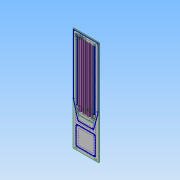
# Autodesk Inventor part: Ply back
Saved by Autodesk Inventor 2013 (Build 170138000, 138)
## iProperties
Created: 2018-07-07
Part Number: Ply back
Material: Generic
Document SubType Name: Modeling
Designer: Jeff Vyduna
Density: 1 g/cm^3
Author: Jeff Vyduna
Autodesk Inventor part; units mm, degrees
ref_plane "YZ Plane" through (0, 0, 0) normal (1, 0, 0) x (0, 1, 0)
ref_plane "XZ Plane" through (0, 0, 0) normal (0, 1, 0) x (-1, 0, 0)
ref_plane "XY Plane" through (0, 0, 0) normal (0, 0, 1) x (1, 0, 0)
sketch "TwoLineColumn" plane through (0, 0, 0) normal (0, 0, 1) x (1, 0, 0)
  line L0 (50.8, -550.7609) -> (50.8, 922.4391) construction
  line L1 (101.6, -550.7609) -> (101.6, 922.4391) construction
  arc A0 (101.6, 922.4391) -> (50.8, 922.4391) centre (76.2, 922.4391) ccw construction
  arc A1 (101.6, -550.7609) -> (152.4, -550.7609) centre (127, -550.7609) ccw construction
  line L2 (56.896, -550.7609) -> (56.896, 922.4391)
  arc A2 (95.504, 922.4391) -> (56.896, 922.4391) centre (76.2, 922.4391) ccw
  line L3 (95.504, 922.4391) -> (95.504, -550.7609)
  arc A3 (95.504, -550.7609) -> (158.496, -550.7609) centre (127, -550.7609) ccw
  line L4 (44.704, -550.7609) -> (44.704, 922.4391)
  arc A4 (107.696, 922.4391) -> (44.704, 922.4391) centre (76.2, 922.4391) ccw
  line L5 (107.696, 922.4391) -> (107.696, -550.7609)
  arc A5 (107.696, -550.7609) -> (146.304, -550.7609) centre (127, -550.7609) ccw
  line L6 (50.8, -550.7609) -> (152.4, -550.7609) construction
  dimension "d4" = 1473.2
  dimension "lineSpacing" = 50.8
  dimension "d6" = 25.4
  dimension "d9" = 6.096
  dimension "d10" = 6.096
  measures "d4" distance of L0.start L0.end
  measures "lineSpacing" distance between parallel lines of L1 L0
  measures "d6" radius of A1
  measures "d9" distance between parallel lines of L1 L3
  measures "d10" distance between parallel lines of L5 L1
sketch "TwoLineColumnEnd" plane through (0, 0, 0) normal (0, 0, 1) x (1, 0, 0)
  line L0 (103.0524, -741.9843) -> (103.0524, 731.2157)
  arc A0 (166.0444, 731.2157) -> (103.0524, 731.2157) centre (134.5484, 731.2157) ccw
  line L1 (166.0444, 731.2157) -> (166.0444, -741.9843)
  line L2 (109.1484, -741.9843) -> (109.1484, 731.2157) construction
  line L3 (159.9484, -741.9843) -> (159.9484, 731.2157) construction
  arc A1 (159.9484, 731.2157) -> (109.1484, 731.2157) centre (134.5484, 731.2157) ccw construction
  line L4 (115.2444, -741.9843) -> (115.2444, 731.2157)
  arc A2 (153.8524, 731.2157) -> (115.2444, 731.2157) centre (134.5484, 731.2157) ccw
  line L5 (153.8524, 731.2157) -> (153.8524, -741.9843)
  line L6 (109.1484, -741.9843) -> (159.9484, -741.9843) construction
  dimension "d22" = 1473.2
  dimension "d23" = 50.8
  dimension "d25" = 6.096
  dimension "d26" = 6.096
  dimension "d29" = 50.8
  measures "d22" distance of L2.start L2.end
  measures "d23" distance between parallel lines of L3 L2
  measures "d25" distance between parallel lines of L3 L5
  measures "d26" distance between parallel lines of L1 L3
  measures "d29" distance of L2.start L6.end
sketch "15mm Neon profile" plane through (0, 0, 0) normal (0, 0, 1) x (1, 0, 0)
  circle A0 centre (522.6685, 24.7098) radius 6.985 construction
  line L0 (516.6995, 21.082) -> (528.6375, 21.082) construction
  line L1 (528.6375, 21.082) -> (528.6375, 6.35) construction
  line L2 (528.6375, 6.35) -> (516.6995, 6.35) construction
  line L3 (516.6995, 6.35) -> (516.6995, 21.082) construction
  point P0 (522.6685, 16.011)
  dimension "d73" = 13.97
  dimension "d74" = 11.938
  dimension "d76" = 14.732
  measures "d73" diameter of A0
  measures "d74" distance of L0.start L0.end
  measures "d76" distance of L0.end L1.end
sketch "U Bolt hole and bore" plane through (0, 0, 0) normal (0, 0, 1) x (1, 0, 0)
  circle A0 centre (40.0435, 30.4025) radius 9.525
  circle A1 centre (74.9685, 30.4025) radius 9.525
  circle A2 centre (40.0435, 30.4025) radius 3.9688
  circle A3 centre (74.9685, 30.4025) radius 3.9688
  point P0 (68.2625, 33.02)
  dimension "d100" = 19.05
  dimension "d102" = 34.925
  dimension "d105" = 7.9375
  measures "d100" diameter of A0
  measures "d102" distance of A1.centre A0.centre
  measures "d105" diameter of A2
sketch "Stock" plane through (0, 0, 0) normal (0, 0, 1) x (1, 0, 0)
  line L0 (0, 0) -> (604.8375, 0)
  line L1 (604.8375, 0) -> (604.8375, 2438.4)
  line L2 (604.8375, 2438.4) -> (0, 2438.4)
  line L3 (0, 2438.4) -> (0, 0)
  dimension "d1" = 604.8375
  dimension "d2" = 2438.4
  constraints: 8 end point, 2 parallel, 1 coincident, 1 horizontal, 1 perpendicular
  measures "d1" distance of L2.end L1.end
  measures "d2" distance of L1.end L0.end
extrude "Stock Extrusion" add sketch "Stock" along normal blind 19.05
sketch "LEDPocket" plane through (0, 0, 19.05) normal (0, 0, 1) x (1, 0, 0)
  line L0 (0, 0) -> (604.8375, 0) projected
  line L1 (604.8375, 0) -> (604.8375, 2438.4) projected
  line L2 (63.5, 120.65) -> (63.5, 0) construction
  line L3 (541.3375, 2438.4) -> (541.3375, 0) construction
  line L4 (68.5882, 922.2642) -> (113.2243, 755.68)
  line L5 (137.7589, 736.854) -> (467.0786, 736.854)
  line L6 (491.6132, 755.68) -> (536.2493, 922.2642)
  line L7 (80.7802, 923.8693) -> (108.8317, 819.18)
  line L8 (133.3662, 800.354) -> (471.4713, 800.354)
  line L9 (496.0058, 819.18) -> (524.0573, 923.8693)
  line L10 (474.1227, 844.55) -> (474.1227, 2317.75)
  arc A0 (537.1147, 2317.75) -> (474.1227, 2317.75) centre (505.6187, 2317.75) ccw
  line L11 (537.1147, 2317.75) -> (537.1147, 928.8382)
  line L12 (480.2187, 844.55) -> (480.2187, 2317.75) construction
  line L13 (531.0187, 844.55) -> (531.0187, 2317.75) construction
  arc A1 (531.0187, 2317.75) -> (480.2187, 2317.75) centre (505.6187, 2317.75) ccw construction
  line L14 (486.3147, 844.55) -> (486.3147, 2317.75)
  arc A2 (524.9227, 2317.75) -> (486.3147, 2317.75) centre (505.6187, 2317.75) ccw
  line L15 (524.9227, 2317.75) -> (524.9227, 930.4433)
  line L16 (480.2187, 844.55) -> (531.0187, 844.55) construction
  line L17 (67.7227, 928.8382) -> (67.7228, 2317.75)
  arc A3 (130.7148, 2317.75) -> (67.7228, 2317.75) centre (99.2188, 2317.75) ccw
  line L18 (130.7148, 2317.75) -> (130.7147, 844.55)
  arc A4 (130.7147, 844.55) -> (169.3227, 844.55) centre (150.0187, 844.55) ccw
  line L19 (73.8187, 844.55) -> (73.8188, 2317.75) construction
  line L20 (124.6187, 844.55) -> (124.6188, 2317.75) construction
  arc A5 (124.6188, 2317.75) -> (73.8188, 2317.75) centre (99.2188, 2317.75) ccw construction
  arc A6 (124.6187, 844.55) -> (175.4187, 844.55) centre (150.0187, 844.55) ccw construction
  line L21 (79.9147, 930.4433) -> (79.9147, 2317.75)
  arc A7 (118.5228, 2317.75) -> (79.9147, 2317.75) centre (99.2188, 2317.75) ccw
  line L22 (118.5228, 2317.75) -> (118.5227, 844.55)
  arc A8 (118.5227, 844.55) -> (181.5147, 844.55) centre (150.0187, 844.55) ccw
  line L23 (73.8187, 844.55) -> (175.4187, 844.55) construction
  line L24 (169.3227, 844.55) -> (169.3228, 2317.75)
  arc A9 (232.3148, 2317.75) -> (169.3228, 2317.75) centre (200.8188, 2317.75) ccw
  line L25 (232.3148, 2317.75) -> (232.3147, 844.55)
  arc A10 (232.3147, 844.55) -> (270.9227, 844.55) centre (251.6187, 844.55) ccw
  line L26 (175.4187, 844.55) -> (175.4188, 2317.75) construction
  line L27 (226.2187, 844.55) -> (226.2188, 2317.75) construction
  arc A11 (226.2188, 2317.75) -> (175.4188, 2317.75) centre (200.8188, 2317.75) ccw construction
  arc A12 (226.2187, 844.55) -> (277.0187, 844.55) centre (251.6187, 844.55) ccw construction
  line L28 (181.5147, 844.55) -> (181.5148, 2317.75)
  arc A13 (220.1227, 2317.75) -> (181.5148, 2317.75) centre (200.8188, 2317.75) ccw
  line L29 (220.1227, 2317.75) -> (220.1227, 844.55)
  arc A14 (220.1227, 844.55) -> (283.1147, 844.55) centre (251.6187, 844.55) ccw
  line L30 (270.9227, 844.55) -> (270.9228, 2317.75)
  arc A15 (333.9148, 2317.75) -> (270.9228, 2317.75) centre (302.4187, 2317.75) ccw
  line L31 (333.9148, 2317.75) -> (333.9147, 844.55)
  arc A16 (333.9147, 844.55) -> (372.5227, 844.55) centre (353.2187, 844.55) ccw
  line L32 (277.0187, 844.55) -> (277.0188, 2317.75) construction
  line L33 (327.8187, 844.55) -> (327.8188, 2317.75) construction
  arc A17 (327.8188, 2317.75) -> (277.0188, 2317.75) centre (302.4187, 2317.75) ccw construction
  arc A18 (327.8187, 844.55) -> (378.6187, 844.55) centre (353.2187, 844.55) ccw construction
  line L34 (283.1147, 844.55) -> (283.1148, 2317.75)
  arc A19 (321.7228, 2317.75) -> (283.1148, 2317.75) centre (302.4187, 2317.75) ccw
  line L35 (321.7228, 2317.75) -> (321.7227, 844.55)
  arc A20 (321.7227, 844.55) -> (384.7148, 844.55) centre (353.2187, 844.55) ccw
  line L36 (372.5227, 844.55) -> (372.5228, 2317.75)
  arc A21 (435.5147, 2317.75) -> (372.5228, 2317.75) centre (404.0188, 2317.75) ccw
  line L37 (435.5147, 2317.75) -> (435.5147, 844.55)
  arc A22 (435.5147, 844.55) -> (474.1227, 844.55) centre (454.8187, 844.55) ccw
  line L38 (378.6187, 844.55) -> (378.6188, 2317.75) construction
  line L39 (429.4187, 844.55) -> (429.4187, 2317.75) construction
  arc A23 (429.4187, 2317.75) -> (378.6188, 2317.75) centre (404.0188, 2317.75) ccw construction
  arc A24 (429.4187, 844.55) -> (480.2187, 844.55) centre (454.8187, 844.55) ccw construction
  line L40 (384.7148, 844.55) -> (384.7148, 2317.75)
  arc A25 (423.3227, 2317.75) -> (384.7148, 2317.75) centre (404.0188, 2317.75) ccw
  line L41 (423.3227, 2317.75) -> (423.3228, 844.55)
  arc A26 (423.3228, 844.55) -> (486.3147, 844.55) centre (454.8187, 844.55) ccw
  arc A27 (67.7227, 928.8382) -> (68.5882, 922.2642) centre (93.1227, 928.8382) ccw
  arc A28 (79.9147, 930.4433) -> (80.7802, 923.8693) centre (105.3147, 930.4433) ccw
  arc A29 (108.8317, 819.18) -> (133.3662, 800.354) centre (133.3662, 825.754) ccw
  arc A30 (471.4713, 800.354) -> (496.0058, 819.18) centre (471.4713, 825.754) ccw
  arc A31 (524.0573, 923.8693) -> (524.9227, 930.4433) centre (499.5227, 930.4433) ccw
  arc A32 (536.2493, 922.2642) -> (537.1147, 928.8382) centre (511.7147, 928.8382) ccw
  arc A33 (467.0786, 736.854) -> (491.6132, 755.68) centre (467.0786, 762.254) ccw
  arc A34 (113.2243, 755.68) -> (137.7589, 736.854) centre (137.7589, 762.254) ccw
  point P0 (0, 2438.4)
  point P1 (67.7227, 925.4942)
  point P2 (537.1147, 925.4942)
  point P3 (79.9147, 927.0993)
  point P4 (524.9227, 927.0993)
  point P5 (113.8761, 800.354)
  point P6 (490.9614, 800.354)
  point P7 (118.2687, 736.854)
  point P8 (486.5687, 736.854)
  point P9 (302.4187, 736.854)
  point P10 (302.4187, 800.354)
  dimension "d7" = 73.8187
  dimension "d18" = 63.5
  dimension "d19" = 120.65
  dimension "d20" = 2438.4
  dimension "d21" = 541.3375
  dimension "d32" = 63.5
  dimension "d33" = 44.196
  dimension "d38" = 844.55
  dimension "d41" = 1473.2
  dimension "d42" = 50.8
  dimension "d43" = 6.096
  dimension "d44" = 6.096
  dimension "d45" = 50.8
  dimension "d49" = 1473.2
  dimension "d50" = 50.8
  dimension "d51" = 25.4
  dimension "d52" = 6.096
  dimension "d53" = 6.096
  dimension "d89" = 120.65
  dimension "d166" = 368.3
  dimension "d167" = 12.192
  dimension "d168" = 25.4
  dimension "d171" = 12.192
  dimension "d172" = 165
  constraints: 80 end point, 70 point on circle, 40 tangent, 35 centre point, 24 vertical, 21 parallel, 16 point on line, 13 equal radius, 12 horizontal alignment, 2 midpoint, 2 perpendicular, 2 vertical alignment, 1 coincident, 1 horizontal, 9 other
  measures "d7" distance from line of L19 point (0, 0)
  measures "d18" distance from line of point (0, 0) L2
  measures "d19" distance of L2.start L2.end
  measures "d20" distance of L3.start L3.end
  measures "d21" distance from line of L0.start L3
  measures "d32" distance between parallel lines of L5 L8
  measures "d33" distance from line of L19.start L8
  measures "d38" distance from line of L19.start L0
  measures "d41" distance of L12.start L12.end
  measures "d42" distance between parallel lines of L13 L12
  measures "d43" distance between parallel lines of L13 L15
  measures "d44" distance between parallel lines of L11 L13
  measures "d45" distance of L12.start L16.end
  measures "d49" distance of L19.start L19.end
  measures "d50" distance between parallel lines of L20 L19
  measures "d51" radius of A6
  measures "d52" distance between parallel lines of L20 L22
  measures "d53" distance between parallel lines of L18 L20
  measures "d89" vertical distance of A3.centre point (0, 2438.4)
  measures "d166" distance of point (118.269, 736.854) point (486.569, 736.854)
  measures "d167" distance between parallel lines of L4 L7
  measures "d168" radius of A27
  measures "d171" distance between parallel lines of L6 L9
  measures "d172" angle of L7 L21
extrude "Main rope pocket" cut sketch "LEDPocket" against normal blind 12.7
sketch "Side profile reference" plane through (0, 0, 0) normal (0, -1, 0) x (1, 0, 0)
  line L0 (0, 0) -> (604.8375, 0) projected
  line L1 (604.8375, 0) -> (604.8375, 19.05) projected
  line L2 (0, 19.05) -> (604.8375, 19.05) projected
  line L3 (0, 0) -> (0, 19.05) projected
  line L4 (598.4875, 38.1) -> (586.2955, 38.1) construction
  line L5 (586.2955, 38.1) -> (586.2955, 25.4) construction
  line L6 (586.2955, 25.4) -> (598.4875, 25.4) construction
  line L7 (598.4875, 25.4) -> (598.4875, 38.1) construction
  line L8 (604.8375, 19.05) -> (541.3375, 19.05) construction
  line L9 (541.3375, 19.05) -> (541.3375, 38.1) construction
  line L10 (541.3375, 38.1) -> (604.8375, 38.1) construction
  line L11 (604.8375, 38.1) -> (604.8375, 19.05) construction
  line L12 (547.6875, 38.1) -> (573.0875, 38.1) construction
  line L13 (573.0875, 38.1) -> (573.0875, 40.64) construction
  line L14 (573.0875, 40.64) -> (547.6875, 40.64) construction
  line L15 (547.6875, 40.64) -> (547.6875, 38.1) construction
  line L16 (579.4375, 40.64) -> (516.6995, 40.64) construction
  line L17 (516.6995, 40.64) -> (516.6995, 45.847) construction
  line L18 (516.6995, 45.847) -> (579.4375, 45.847) construction
  line L19 (579.4375, 45.847) -> (579.4375, 40.64) construction
  circle A0 centre (522.6685, 24.7098) radius 6.985 construction
  line L20 (516.6995, 21.082) -> (528.6375, 21.082) construction
  line L21 (528.6375, 21.082) -> (528.6375, 6.35) construction
  line L22 (528.6375, 6.35) -> (516.6995, 6.35) construction
  line L23 (516.6995, 6.35) -> (516.6995, 21.082) construction
  circle A1 centre (592.3915, 43.7598) radius 6.985 construction
  line L24 (586.4225, 40.132) -> (598.3605, 40.132) construction
  line L25 (598.3605, 40.132) -> (598.3605, 25.4) construction
  line L26 (598.3605, 25.4) -> (586.4225, 25.4) construction
  line L27 (586.4225, 25.4) -> (586.4225, 40.132) construction
  point P0 (566.7375, 19.05)
  point P1 (592.3915, 25.4)
  point P2 (592.3915, 25.4)
  dimension "d75" = 12.7
  dimension "d80" = 12.192
  dimension "d88" = 6.35
  dimension "d90" = 63.5
  dimension "d91" = 19.05
  dimension "d92" = 25.4
  dimension "d93" = 2.54
  dimension "d94" = 6.35
  dimension "d95" = 12.7
  dimension "d96" = 6.35
  dimension "d97" = 5.207
  dimension "d98" = 0
  dimension "d99" = 12.7
  constraints: 32 end point, 8 parallel, 5 horizontal, 4 perpendicular, 1 coincident, 1 collinear, 1 midpoint, 1 point on line, 1 other
  measures "d80" distance of L6.end L5.end
  measures "d88" horizontal distance of L1.end L6.end
  measures "d90" distance of L9.end L10.end
  measures "d91" distance of L8.end L9.end
  measures "d92" distance of L14.end L13.end
  measures "d93" distance of L13.end L12.end
  measures "d94" distance of L9.end L12.start
  measures "d96" horizontal distance of L16.start L12.end
  measures "d97" distance of L16.end L17.end
  measures "d99" vertical distance of L10.end L6.end
sketch "U-Bolt holes" plane through (0, 0, 19.05) normal (0, 0, 1) x (1, 0, 0)
  line L0 (0, 0) -> (604.8375, 0) projected
  line L1 (604.8375, 0) -> (604.8375, 2438.4) projected
  line L2 (0, 2438.4) -> (0, 0) projected
  line L3 (604.8375, 2438.4) -> (0, 2438.4) projected
  point P0 (53.975, 33.02)
  point P1 (88.9, 33.02)
  point P2 (515.9375, 33.02)
  point P3 (550.8625, 33.02)
  point P4 (531.8125, 2365.375)
  point P5 (496.8875, 2365.375)
  point P6 (73.025, 2365.375)
  point P7 (107.95, 2365.375)
  dimension "d109" = 33.02
  dimension "d110" = 34.925
  dimension "d111" = 34.925
  dimension "d112" = 19.05
  dimension "d113" = 53.975
  dimension "d114" = 53.975
  dimension "d115" = 34.925
  dimension "d116" = 34.925
  dimension "d117" = 19.05
  dimension "d126" = 73.025
  constraints: 6 horizontal alignment
  measures "d109" distance from line of L0 point (53.975, 33.02)
  measures "d110" distance of point (88.9, 33.02) point (53.975, 33.02)
  measures "d111" distance of point (550.862, 33.02) point (515.937, 33.02)
  measures "d112" horizontal distance of point (53.975, 33.02) point (73.025, 2365.375)
  measures "d113" distance from line of L1 point (550.862, 33.02)
  measures "d114" distance from line of L2 point (53.975, 33.02)
  measures "d115" distance of point (73.025, 2365.375) point (107.95, 2365.375)
  measures "d116" distance of point (531.812, 2365.375) point (496.887, 2365.375)
  measures "d117" horizontal distance of point (531.812, 2365.375) point (550.862, 33.02)
  measures "d126" distance from line of L3 point (73.025, 2365.375)
hole "Hole1" at (73.025, 2365.375, 19.05) at (107.95, 2365.375, 19.05) at (496.8875, 2365.375, 19.05) at (531.8125, 2365.375, 19.05) at (550.8625, 33.02, 19.05) at (515.9375, 33.02, 19.05) at (88.9, 33.02, 19.05) at (53.975, 33.02, 19.05) direction (0, 0, -1) diameter 7.9375 end through all counterbore diameter 19.05 counterbore depth 6.35
ref_plane "Work Plane1" through (0, 0, 6.35) normal (0, 0, 1) x (1, 0, 0)
sketch "WeatherProof panel" plane through (0, 0, 6.35) normal (0, 0, 1) x (1, 0, 0)
  line L0 (524.9228, 801.1635) -> (524.9227, 2317.75) projected
  line L1 (370.9352, 749.554) -> (418.5602, 749.554)
  line L2 (423.3227, 744.7915) -> (423.3227, 709.8665)
  line L3 (418.5602, 705.104) -> (370.9352, 705.104)
  line L4 (366.1727, 709.8665) -> (366.1727, 744.7915)
  arc A0 (370.9352, 749.554) -> (366.1727, 744.7915) centre (370.9352, 744.7915) ccw
  arc A1 (366.1727, 709.8665) -> (370.9352, 705.104) centre (370.9352, 709.8665) ccw
  arc A2 (423.3227, 744.7915) -> (418.5602, 749.554) centre (418.5602, 744.7915) ccw
  arc A3 (418.5602, 705.104) -> (423.3227, 709.8665) centre (418.5602, 709.8665) ccw
  line L5 (116.0705, 749.554) -> (488.767, 749.554) projected
  point P0 (105.3147, 749.554)
  point P1 (524.9227, 774.954)
  point P2 (499.5227, 749.554)
  point P3 (0, 0)
  point P4 (423.3227, 705.104)
  point P5 (423.3227, 749.554)
  point P6 (366.1727, 705.104)
  point P7 (524.9228, 796.1544)
  point P8 (99.0385, 749.554)
  point P9 (505.799, 749.554)
  dimension "d127" = 44.45
  dimension "d129" = 57.15
  dimension "d130" = 4.7625
  dimension "d131" = 101.6
  constraints: 8 end point, 8 point on circle, 8 tangent, 6 point on line, 4 centre point, 3 equal radius, 2 parallel, 1 collinear, 1 horizontal, 1 perpendicular
  measures "d127" distance of point (423.323, 749.554) point (423.323, 705.104)
  measures "d129" distance of point (423.323, 705.104) point (366.173, 705.104)
  measures "d130" radius of A0
  measures "d131" distance between parallel lines of L0 L2
extrude "Through Panel Extrusion5" cut sketch "WeatherProof panel" against normal through all
sketch "Exclaim Point" plane through (0, 0, 19.05) normal (0, 0, 1) x (1, 0, 0)
  circle A0 centre (88.9, 33.02) radius 9.525 projected
  circle A1 centre (550.8625, 33.02) radius 9.525 projected
  circle A2 centre (496.8875, 2365.375) radius 9.525 construction
  circle A3 centre (73.025, 2365.375) radius 9.525 construction
  circle A4 centre (107.95, 2365.375) radius 9.525 construction
  circle A5 centre (531.8125, 2365.375) radius 9.525 construction
  circle A6 centre (515.9375, 33.02) radius 9.525 projected
  circle A7 centre (53.975, 33.02) radius 9.525 projected
  line L0 (0, 0) -> (604.8375, 0) projected
  line L1 (604.8375, 0) -> (604.8375, 2438.4) projected
  line L2 (604.8375, 2438.4) -> (0, 2438.4) projected
  line L3 (0, 2438.4) -> (0, 0) projected
  line L4 (63.5, 2374.9) -> (541.3375, 2374.9) construction
  line L5 (541.3375, 2374.9) -> (541.3375, 63.5) construction
  line L6 (541.3375, 63.5) -> (63.5, 63.5) construction
  line L7 (63.5, 63.5) -> (63.5, 2374.9) construction
  line L8 (10.414, 2408.936) -> (10.414, 1022.3815) construction
  line L9 (11.0631, 1017.451) -> (115.5252, 627.593) construction
  line L10 (133.9261, 613.4735) -> (470.9114, 613.4735) construction
  line L11 (489.3123, 627.593) -> (593.7744, 1017.451) construction
  line L12 (594.4235, 1022.3815) -> (594.4235, 2408.936) construction
  line L13 (575.3735, 2427.986) -> (29.464, 2427.986) construction
  line L14 (127, 477.8375) -> (477.8375, 477.8375) construction
  line L15 (477.8375, 477.8375) -> (477.8375, 127) construction
  line L16 (477.8375, 127) -> (127, 127) construction
  line L17 (127, 127) -> (127, 477.8375) construction
  line L18 (63.5, 541.3375) -> (541.3375, 541.3375) construction
  line L19 (99.314, 524.5735) -> (505.5235, 524.5735) construction
  line L20 (524.5735, 505.5235) -> (524.5735, 99.314) construction
  line L21 (505.5235, 80.264) -> (99.314, 80.264) construction
  line L22 (80.264, 99.314) -> (80.264, 505.5235) construction
  arc A8 (524.5735, 505.5235) -> (505.5235, 524.5735) centre (505.5235, 505.5235) ccw construction
  arc A9 (99.314, 524.5735) -> (80.264, 505.5235) centre (99.314, 505.5235) ccw construction
  arc A10 (80.264, 99.314) -> (99.314, 80.264) centre (99.314, 99.314) ccw construction
  arc A11 (505.5235, 80.264) -> (524.5735, 99.314) centre (505.5235, 99.314) ccw construction
  line L23 (505.5235, 520.5095) -> (99.314, 520.5095)
  arc A12 (99.314, 520.5095) -> (84.328, 505.5235) centre (99.314, 505.5235) ccw
  line L24 (84.328, 505.5235) -> (84.328, 99.314)
  arc A13 (84.328, 99.314) -> (99.314, 84.328) centre (99.314, 99.314) ccw
  line L25 (99.314, 84.328) -> (505.5235, 84.328)
  arc A14 (505.5235, 84.328) -> (520.5095, 99.314) centre (505.5235, 99.314) ccw
  line L26 (520.5095, 99.314) -> (520.5095, 505.5235)
  arc A15 (520.5095, 505.5235) -> (505.5235, 520.5095) centre (505.5235, 505.5235) ccw
  line L27 (505.5235, 528.6375) -> (99.314, 528.6375)
  arc A16 (99.314, 528.6375) -> (76.2, 505.5235) centre (99.314, 505.5235) ccw
  line L28 (76.2, 505.5235) -> (76.2, 99.314)
  arc A17 (76.2, 99.314) -> (99.314, 76.2) centre (99.314, 99.314) ccw
  line L29 (99.314, 76.2) -> (505.5235, 76.2)
  arc A18 (505.5235, 76.2) -> (528.6375, 99.314) centre (505.5235, 99.314) ccw
  line L30 (528.6375, 99.314) -> (528.6375, 505.5235)
  arc A19 (528.6375, 505.5235) -> (505.5235, 528.6375) centre (505.5235, 505.5235) ccw
  arc A20 (29.464, 2427.986) -> (10.414, 2408.936) centre (29.464, 2408.936) ccw construction
  arc A21 (594.4235, 2408.936) -> (575.3735, 2427.986) centre (575.3735, 2408.936) ccw construction
  arc A22 (593.7744, 1017.451) -> (594.4235, 1022.3815) centre (575.3735, 1022.3815) ccw construction
  arc A23 (470.9114, 613.4735) -> (489.3123, 627.593) centre (470.9114, 632.5235) ccw construction
  arc A24 (115.5252, 627.593) -> (133.9261, 613.4735) centre (133.9261, 632.5235) ccw construction
  arc A25 (10.414, 1022.3815) -> (11.0631, 1017.451) centre (29.464, 1022.3815) ccw construction
  line L31 (589.8489, 1018.5028) -> (485.3867, 628.6448)
  arc A26 (470.9114, 617.5375) -> (485.3867, 628.6448) centre (470.9114, 632.5235) ccw
  line L32 (470.9114, 617.5375) -> (133.9261, 617.5375)
  arc A27 (119.4508, 628.6448) -> (133.9261, 617.5375) centre (133.9261, 632.5235) ccw
  line L33 (119.4508, 628.6448) -> (14.9886, 1018.5028)
  arc A28 (14.478, 1022.3815) -> (14.9886, 1018.5028) centre (29.464, 1022.3815) ccw
  line L34 (14.478, 1022.3815) -> (14.478, 2408.936)
  arc A29 (29.464, 2423.922) -> (14.478, 2408.936) centre (29.464, 2408.936) ccw
  line L35 (29.464, 2423.922) -> (575.3735, 2423.922)
  arc A30 (590.3595, 2408.936) -> (575.3735, 2423.922) centre (575.3735, 2408.936) ccw
  line L36 (590.3595, 2408.936) -> (590.3595, 1022.3815)
  arc A31 (589.8489, 1018.5028) -> (590.3595, 1022.3815) centre (575.3735, 1022.3815) ccw
  line L37 (597.6999, 1016.3991) -> (493.2378, 626.5412)
  arc A32 (470.9114, 609.4095) -> (493.2378, 626.5412) centre (470.9114, 632.5235) ccw
  line L38 (470.9114, 609.4095) -> (133.9261, 609.4095)
  arc A33 (111.5997, 626.5412) -> (133.9261, 609.4095) centre (133.9261, 632.5235) ccw
  line L39 (111.5997, 626.5412) -> (7.1376, 1016.3991)
  arc A34 (6.35, 1022.3815) -> (7.1376, 1016.3991) centre (29.464, 1022.3815) ccw
  line L40 (6.35, 1022.3815) -> (6.35, 2408.936)
  arc A35 (29.464, 2432.05) -> (6.35, 2408.936) centre (29.464, 2408.936) ccw
  line L41 (29.464, 2432.05) -> (575.3735, 2432.05)
  arc A36 (598.4875, 2408.936) -> (575.3735, 2432.05) centre (575.3735, 2408.936) ccw
  line L42 (598.4875, 2408.936) -> (598.4875, 1022.3815)
  arc A37 (597.6999, 1016.3991) -> (598.4875, 1022.3815) centre (575.3735, 1022.3815) ccw
  line L43 (63.5, 645.2235) -> (541.3375, 645.2235) construction
  line L44 (541.3375, 581.7235) -> (63.5, 581.7235) construction
  line L45 (63.5, 645.2235) -> (127, 645.2235) construction
  line L46 (127, 645.2235) -> (127, 848.4235) construction
  line L47 (127, 848.4235) -> (63.5, 848.4235) construction
  line L48 (63.5, 848.4235) -> (63.5, 645.2235) construction
  line L49 (541.3375, 645.2235) -> (477.8375, 645.2235) construction
  line L50 (477.8375, 645.2235) -> (477.8375, 848.4235) construction
  line L51 (477.8375, 848.4235) -> (541.3375, 848.4235) construction
  line L52 (541.3375, 848.4235) -> (541.3375, 645.2235) construction
  point P0 (10.414, 1019.8735)
  point P1 (485.5289, 613.4735)
  point P2 (594.4235, 1019.8735)
  dimension "d138" = 63.5
  dimension "d139" = 10.414
  dimension "d140" = 10.414
  dimension "d141" = 10.414
  dimension "d142" = 165
  dimension "d144" = 63.5
  dimension "d145" = 63.5
  dimension "d146" = 63.5
  dimension "d147" = 63.5
  dimension "d148" = 16.764
  dimension "d149" = 16.764
  dimension "d150" = 16.764
  dimension "d151" = 88.9
  dimension "d152" = 406.4
  dimension "d154" = 19.05
  dimension "d155" = 19.05
  dimension "d156" = 4.064
  dimension "d157" = 8.128
  dimension "d158" = 19.05
  dimension "d159" = 4.064
  dimension "d160" = 8.128
  dimension "d161" = 63.5
  dimension "d162" = 31.75
  dimension "d163" = 63.5
  dimension "d164" = 203.2
  dimension "d165" = 63.5
  constraints: 98 end point, 60 point on circle, 30 centre point, 20 tangent, 14 parallel, 12 point on line, 11 perpendicular, 7 equal radius, 4 equal length, 4 horizontal, 1 horizontal alignment, 39 other
  measures "d138" distance between parallel lines of L1 L5
  measures "d139" distance between parallel lines of L3 L8
  measures "d140" distance between parallel lines of L2 L13
  measures "d141" distance between parallel lines of L1 L12
  measures "d142" angle of L9 L8
  measures "d144" distance between parallel lines of L17 L7
  measures "d145" distance between parallel lines of L6 L16
  measures "d146" distance between parallel lines of L5 L15
  measures "d147" distance between parallel lines of L18 L14
  measures "d148" distance between parallel lines of L7 L22
  measures "d149" distance between parallel lines of L18 L19
  measures "d150" distance between parallel lines of L5 L20
  measures "d151" distance between parallel lines of L19 L10
  measures "d152" vertical distance of point (485.529, 613.474) point (594.423, 1019.874)
  measures "d154" radius of A8
  measures "d155" radius of A9
  measures "d156" distance between parallel lines of L27 L19
  measures "d157" distance between parallel lines of L23 L27
  measures "d158" radius of A20
  measures "d159" distance between parallel lines of L13 L41
  measures "d160" distance between parallel lines of L35 L41
  measures "d161" distance between parallel lines of L44 L43
  measures "d162" distance between parallel lines of L43 L10
  measures "d163" distance of L47.end L46.end
  measures "d164" distance of L46.end L45.end
  measures "d165" distance of L50.end L51.end
sketch "Sketch11" plane through (0, 0, 19.05) normal (0, 0, 1) x (1, 0, 0)
  circle A0 centre (88.9, 33.02) radius 9.525 projected
  circle A1 centre (550.8625, 33.02) radius 9.525 projected
  circle A2 centre (496.8875, 2365.375) radius 9.525 projected
  circle A3 centre (73.025, 2365.375) radius 9.525 projected
  circle A4 centre (107.95, 2365.375) radius 9.525 projected
  circle A5 centre (531.8125, 2365.375) radius 9.525 projected
  circle A6 centre (515.9375, 33.02) radius 9.525 projected
  circle A7 centre (53.975, 33.02) radius 9.525 projected
  line L0 (0, 0) -> (604.8375, 0) projected
  line L1 (604.8375, 0) -> (604.8375, 2438.4) projected
  line L2 (604.8375, 2438.4) -> (0, 2438.4) projected
  line L3 (0, 2438.4) -> (0, 0) projected
  arc A8 (435.5147, 844.55) -> (474.1227, 844.55) centre (454.8187, 844.55) ccw projected
  line L4 (474.1227, 844.55) -> (474.1227, 2317.75) projected
  arc A9 (537.1147, 2317.75) -> (474.1227, 2317.75) centre (505.6187, 2317.75) ccw projected
  line L5 (537.1147, 2317.75) -> (537.1147, 928.8382) projected
  arc A10 (536.2493, 922.2642) -> (537.1147, 928.8382) centre (511.7147, 928.8382) ccw projected
  line L6 (536.2493, 922.2642) -> (491.6132, 755.68) projected
  arc A11 (467.0786, 736.854) -> (491.6132, 755.68) centre (467.0786, 762.254) ccw projected
  line L7 (467.0786, 736.854) -> (137.7589, 736.854) projected
  arc A12 (113.2243, 755.68) -> (137.7589, 736.854) centre (137.7589, 762.254) ccw projected
  line L8 (113.2243, 755.68) -> (68.5882, 922.2642) projected
  arc A13 (67.7227, 928.8382) -> (68.5882, 922.2642) centre (93.1227, 928.8382) ccw projected
  line L9 (67.7227, 928.8382) -> (67.7228, 2317.75) projected
  arc A14 (130.7148, 2317.75) -> (67.7228, 2317.75) centre (99.2188, 2317.75) ccw projected
  line L10 (130.7148, 2317.75) -> (130.7147, 844.55) projected
  arc A15 (130.7147, 844.55) -> (169.3227, 844.55) centre (150.0187, 844.55) ccw projected
  line L11 (169.3227, 844.55) -> (169.3228, 2317.75) projected
  arc A16 (232.3148, 2317.75) -> (169.3228, 2317.75) centre (200.8188, 2317.75) ccw projected
  line L12 (232.3148, 2317.75) -> (232.3147, 844.55) projected
  arc A17 (232.3147, 844.55) -> (270.9227, 844.55) centre (251.6187, 844.55) ccw projected
  line L13 (270.9227, 844.55) -> (270.9228, 2317.75) projected
  arc A18 (333.9148, 2317.75) -> (270.9228, 2317.75) centre (302.4187, 2317.75) ccw projected
  line L14 (333.9148, 2317.75) -> (333.9147, 844.55) projected
  arc A19 (333.9147, 844.55) -> (372.5227, 844.55) centre (353.2187, 844.55) ccw projected
  line L15 (372.5227, 844.55) -> (372.5228, 2317.75) projected
  arc A20 (435.5147, 2317.75) -> (372.5228, 2317.75) centre (404.0188, 2317.75) ccw projected
  line L16 (435.5147, 2317.75) -> (435.5147, 844.55) projected
  line L17 (143.6687, 844.55) -> (143.6687, 2317.75)
  line L18 (156.3687, 2317.75) -> (156.3687, 844.55)
  arc A21 (156.3687, 2317.75) -> (143.6687, 2317.75) centre (150.0187, 2317.75) ccw
  arc A22 (143.6687, 844.55) -> (156.3687, 844.55) centre (150.0187, 844.55) ccw
  line L19 (194.4687, 844.55) -> (194.4687, 2317.75)
  line L20 (207.1687, 2317.75) -> (207.1687, 844.55)
  arc A23 (207.1687, 2317.75) -> (194.4687, 2317.75) centre (200.8187, 2317.75) ccw
  arc A24 (194.4687, 844.55) -> (207.1687, 844.55) centre (200.8187, 844.55) ccw
  line L21 (245.2687, 844.55) -> (245.2687, 2317.75)
  line L22 (257.9687, 2317.75) -> (257.9687, 844.55)
  arc A25 (257.9687, 2317.75) -> (245.2687, 2317.75) centre (251.6187, 2317.75) ccw
  arc A26 (245.2687, 844.55) -> (257.9687, 844.55) centre (251.6187, 844.55) ccw
  line L23 (296.0687, 844.55) -> (296.0687, 2317.75)
  line L24 (308.7687, 2317.75) -> (308.7687, 844.55)
  arc A27 (308.7687, 2317.75) -> (296.0687, 2317.75) centre (302.4187, 2317.75) ccw
  arc A28 (296.0687, 844.55) -> (308.7687, 844.55) centre (302.4187, 844.55) ccw
  line L25 (346.8687, 844.55) -> (346.8687, 2317.75)
  line L26 (359.5687, 2317.75) -> (359.5687, 844.55)
  arc A29 (359.5687, 2317.75) -> (346.8687, 2317.75) centre (353.2187, 2317.75) ccw
  arc A30 (346.8687, 844.55) -> (359.5687, 844.55) centre (353.2187, 844.55) ccw
  line L27 (397.6687, 844.55) -> (397.6687, 2317.75)
  line L28 (410.3687, 2317.75) -> (410.3687, 844.55)
  arc A31 (410.3687, 2317.75) -> (397.6687, 2317.75) centre (404.0187, 2317.75) ccw
  arc A32 (397.6687, 844.55) -> (410.3687, 844.55) centre (404.0187, 844.55) ccw
  line L29 (448.4687, 844.55) -> (448.4687, 2317.75)
  line L30 (461.1687, 2317.75) -> (461.1687, 844.55)
  arc A33 (461.1687, 2317.75) -> (448.4687, 2317.75) centre (454.8187, 2317.75) ccw
  arc A34 (448.4687, 844.55) -> (461.1687, 844.55) centre (454.8187, 844.55) ccw
  line L31 (92.8688, 928.8382) -> (92.8687, 2317.75)
  line L32 (105.5687, 2317.75) -> (105.5688, 928.8382)
  arc A35 (105.5687, 2317.75) -> (92.8687, 2317.75) centre (99.2188, 2317.75) ccw
  arc A36 (92.8688, 928.8382) -> (105.5688, 928.8382) centre (99.2188, 928.8382) ccw
  arc A37 (499.2688, 928.8382) -> (511.9688, 928.8382) centre (505.6187, 928.8382) ccw
  line L33 (499.2688, 928.8382) -> (499.2687, 2317.75)
  line L34 (511.9688, 2317.75) -> (511.9688, 928.8382)
  arc A38 (511.9688, 2317.75) -> (499.2687, 2317.75) centre (505.6187, 2317.75) ccw
  point P0 (499.5227, 928.8382)
  dimension "d173" = 12.7
  dimension "d176" = 50.8
  dimension "d181" = 12.7
  dimension "d184" = 406.4
  constraints: 36 end point, 36 point on circle, 18 centre point, 8 tangent, 2 coincident, 2 horizontal, 2 horizontal alignment, 2 parallel, 2 vertical, 71 other
  measures "d173" distance of L17.end L18.start
  measures "d176" distance of L18.start L20.start
  measures "d181" distance of L31.end L32.start
  measures "d184" distance of L32.end L34.end
equation "\"d7\" = -4.5 * lineSpacing + 0.5 * signW"
equation "\"d18\" = borderW"
equation "\"d4\" = litH"
equation "\"d6\" = 0.5 * lineSpacing"
equation "\"d9\" = 0.5 * pathW"
equation "\"d10\" = 0.5 * pathW"
equation "\"d22\" = litH"
equation "\"d25\" = 0.5 * pathW"
equation "\"d26\" = 0.5 * pathW"
equation "\"d29\" = lineSpacing"
equation "\"d1\" = signW"
equation "\"d2\" = signH"
equation "\"d20\" = signH"
equation "\"d21\" = signW - borderW"
equation "\"d32\" = ePocketH"
equation "\"d33\" = litHClearanceH"
equation "\"d45\" = d47"
equation "\"d51\" = 0.5 * d50"
equation "\"litH\" = 1473.2"
equation "\"borderW\" = 63.5"
equation "\"pathEndMillD\" = 9.525"
equation "\"signW\" = -0.5 * pathEndMillD + 0.5 * ply4x8w"
equation "\"pathW\" = 12.192"
equation "\"ply4x8w\" = 1219.2"
equation "\"signH\" = 2438.4"
equation "\"ePocketH\" = 63.5"
equation "\"minBendR\" = 25.4"
equation "\"outlineCOffset\" = 10.414"
equation "\"sRopeChannel\" = 8.128"
equation "\"sRopeDepth\" = 10.922"
equation "\"sRopeBendR\" = 19.05"
equation "\"litHClearanceH\" = 44.196"
equation "\"d47\" = 50.8"
body "Solid1"
